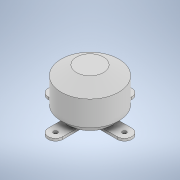
# Autodesk Inventor part: Motor
Saved by Autodesk Inventor 2020 (Build 240168000, 168)
## iProperties
Created: 2019-09-24
Part Number: Motor
Material: Generic
Document SubType Name: Modeling
Designer: User
Density: 1 g/cm^3
Appearance: Default
Author: User
Autodesk Inventor part; units mm, degrees
ref_plane "YZ Plane" through (0, 0, 0) normal (1, 0, 0) x (0, 1, 0)
ref_plane "XZ Plane" through (0, 0, 0) normal (0, 1, 0) x (-1, 0, 0)
ref_plane "XY Plane" through (0, 0, 0) normal (0, 0, 1) x (1, 0, 0)
sketch "Sketch1" plane through (0, 0, 0) normal (0, 0, 1) x (1, 0, 0)
  line L0 (0, 0) -> (17.78, 0)
  line L1 (17.78, 0) -> (22.987, 5.588)
  line L2 (22.987, 5.588) -> (22.987, 25.527)
  line L3 (22.987, 25.527) -> (10.795, 33.02)
  line L4 (10.795, 33.02) -> (0, 33.02)
  line L5 (0, 33.02) -> (0, 0)
  dimension "d0" = 17.78
  dimension "d1" = 33.02
  dimension "d2" = 22.987
  dimension "d3" = 5.588
  dimension "d4" = 19.939
  dimension "d5" = 10.795
  constraints: 12 end point, 2 perpendicular, 1 horizontal, 1 parallel
  measures "d0" distance of L0.start L0.end
  measures "d1" distance between parallel lines of L0 L4
  measures "d2" distance between parallel lines of L5 L2
  measures "d3" distance from line of L0 L1.end
  measures "d4" distance of L1.end L2.end
  measures "d5" distance of L3.end L4.end
revolve "Revolution1" add sketch "Sketch1" angle 360 about axis through (0, 33.02, 0) along (0, -1, 0)
sketch "Sketch2" plane through (0, 0, 0) normal (0, -1, 0) x (1, 0, 0)
  line L0 (0, 27.5971) -> (0, -27.5971) construction
  line L1 (-5.9055, 27.5971) -> (-5.9055, -27.5971)
  line L2 (5.9055, -27.5971) -> (5.9055, 27.5971)
  arc A0 (5.9055, 27.5971) -> (-5.9055, 27.5971) centre (0, 27.5971) ccw
  arc A1 (-5.9055, -27.5971) -> (5.9055, -27.5971) centre (0, -27.5971) ccw
  line L3 (-27.5971, 0) -> (27.5971, 0) construction
  line L4 (-27.5971, 5.9055) -> (27.5971, 5.9055)
  line L5 (27.5971, -5.9055) -> (-27.5971, -5.9055)
  arc A2 (-27.5971, 5.9055) -> (-27.5971, -5.9055) centre (-27.5971, 0) ccw
  arc A3 (27.5971, -5.9055) -> (27.5971, 5.9055) centre (27.5971, 0) ccw
  circle A4 centre (27.5971, 0) radius 1.6193
  circle A5 centre (0, -27.5971) radius 1.6193
  circle A6 centre (-27.5971, 0) radius 1.6193
  circle A7 centre (0, 27.5971) radius 1.6193
  point P0 (0, 0)
  point P1 (5.9055, 5.9055)
  point P2 (-5.9055, 5.9055)
  point P3 (-5.9055, -5.9055)
  point P4 (5.9055, -5.9055)
  dimension "d7" = 11.811
  dimension "d8" = 55.1942
  dimension "d9" = 3.2385
  constraints: 16 end point, 8 centre point, 8 point on circle, 8 tangent, 4 coincident, 4 equal radius, 2 midpoint, 2 parallel, 2 perpendicular, 1 vertical
  measures "d7" distance between parallel lines of L5 L4
  measures "d8" distance of L5.start L5.end
  measures "d9" diameter of A7
extrude "Extrusion1" add sketch "Sketch2" along normal blind 1.9304
body "Solid1"
